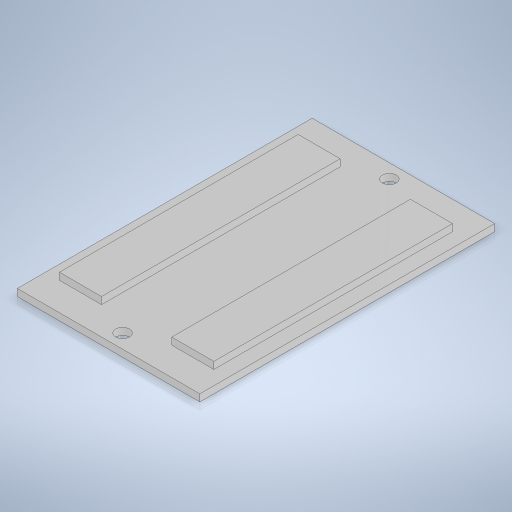
# Autodesk Inventor part: 1011
Saved by Autodesk Inventor 2024 (Build 280153000, 153)
## iProperties
Created: 2024-07-12
Part Number: 1011
Material: Aluminum 6061-AHC
Document SubType Name: Modeling
Designer: ffogue
Density: 2.7 g/cm^3
Appearance: Aluminium - dunkel
Author: ffogue
Autodesk Inventor part; units mm, degrees
ref_plane "YZ Plane" through (0, 0, 0) normal (1, 0, 0) x (0, 1, 0)
ref_plane "XZ Plane" through (0, 0, 0) normal (0, 1, 0) x (-1, 0, 0)
ref_plane "XY Plane" through (0, 0, 0) normal (0, 0, 1) x (1, 0, 0)
sketch "Skizze1" plane through (0, 0, 0) normal (0, 0, 1) x (1, 0, 0)
  line L0 (0, 0) -> (52, 0)
  line L1 (52, 0) -> (52, -84)
  line L2 (52, -84) -> (0, -84)
  line L3 (0, -84) -> (0, 0)
  dimension "d0" = 52
  dimension "d1" = 84
  constraints: 8 end point, 2 parallel, 1 horizontal, 1 perpendicular
  measures "d0" distance between parallel lines of L3 L1
  measures "d1" distance between parallel lines of L2 L0
extrude "Extrusion1" add sketch "Skizze1" along normal blind 2
sketch "Skizze2" plane through (0, 0, 2) normal (0, 0, 1) x (1, 0, 0)
  line L0 (48, -8) -> (4, -8)
  line L1 (4, -8) -> (4, -76)
  line L2 (4, -76) -> (48, -76)
  line L3 (48, -76) -> (48, -8)
  line L4 (52, 0) -> (0, 0) projected
  line L5 (52, -84) -> (52, 0) projected
  line L6 (0, -84) -> (52, -84) projected
  point P0 (26, -8)
  point P1 (26, 0)
  dimension "d4" = 4
  dimension "d5" = 8
  dimension "d6" = 8
  constraints: 8 end point, 2 midpoint, 2 parallel, 1 horizontal, 1 perpendicular, 1 vertical alignment
  measures "d4" distance between parallel lines of L3 L5
  measures "d5" distance between parallel lines of L0 L4
  measures "d6" distance between parallel lines of L6 L2
extrude "Extrusion2" add sketch "Skizze2" along normal blind 2
sketch "Skizze3" plane through (4, -8, 2) normal (0, 1, 0) x (1, 0, 0)
  line L0 (48, 2) -> (-4, 2) projected
  line L1 (-4, 2) -> (-4, 0) projected
  line L2 (48, 0) -> (-4, 0) projected
  line L3 (48, 2) -> (48, 0) projected
  line L4 (44, -2) -> (0, -2) projected
  line L5 (32, 0) -> (12, 0)
  line L6 (12, 0) -> (12, -2)
  line L7 (12, -2) -> (32, -2)
  line L8 (32, -2) -> (32, 0)
  line L9 (44, 0) -> (44, -2) projected
  point P0 (44, -1)
  point P1 (32, -2)
  point P2 (12, 0)
  dimension "d9" = 20
  dimension "d10" = 12
  constraints: 8 end point, 2 parallel, 2 point on line, 1 horizontal, 1 midpoint, 1 perpendicular
  measures "d9" distance between parallel lines of L6 L8
  measures "d10" distance from line of L8 point (44, -1)
extrude "Extrusion3" cut sketch "Skizze3" against normal through all contours L2 L8 L4 L6
sketch "Skizze4" plane through (0, 0, 2) normal (0, 0, 1) x (1, 0, 0)
  line L0 (52, 0) -> (0, 0) projected
  line L1 (0, -84) -> (52, -84) projected
  point P0 (26, -4)
  point P1 (26, -80)
  point P2 (26, 0)
  dimension "d20" = 4
  dimension "d21" = 4
  constraints: 2 vertical alignment, 1 midpoint
  measures "d20" distance from line of point (26, -4) L0
  measures "d21" distance from line of L1 point (26, -80)
hole "Bohrung1" at (26, -4, 2) at (26, -80, 2) direction (0, 0, -1) diameter 4 depth 2
equation "\"d6\" = d5"
equation "\"d21\" = d20"
